Autodesk Inventor part; units mm, degrees
(part 2 of 2)
  spline S259 degree 2 poles (-78.2039, 3.4527) (-78.362, 3.5738) (-78.5473, 3.9615) (-78.5473, 4.2678) knots 0 0 0 1 2 2 2
  spline S260 degree 2 poles (-78.5473, 4.2678) (-78.5473, 4.5074) (-78.3842, 4.91) (-78.236, 5.0582) knots 0 0 0 1 2 2 2
  spline S261 degree 2 poles (-78.236, 5.0582) (-78.0878, 5.2064) (-77.6581, 5.3744) (-77.3938, 5.3744) knots 0 0 0 1 2 2 2
  spline S262 degree 2 poles (-77.3938, 5.3744) (-77.127, 5.3744) (-76.7145, 5.2262) (-76.5663, 5.0706) knots 0 0 0 1 2 2 2
  spline S263 degree 2 poles (-76.5663, 5.0706) (-76.3934, 4.8977) (-76.2156, 4.3493) (-76.2156, 3.9591) knots 0 0 0 1 2 2 2
  spline S264 degree 2 poles (-76.9739, 4.0727) (-76.9739, 4.3222) (-77.0579, 4.6433) (-77.1344, 4.7322) knots 0 0 0 1 2 2 2
  spline S265 degree 2 poles (-77.1344, 4.7322) (-77.1863, 4.7989) (-77.3197, 4.8557) (-77.3962, 4.8557) knots 0 0 0 1 2 2 2
  spline S266 degree 2 poles (-77.3962, 4.8557) (-77.4654, 4.8557) (-77.5938, 4.8014) (-77.6531, 4.7322) knots 0 0 0 1 2 2 2
  spline S267 degree 2 poles (-77.6531, 4.7322) (-77.705, 4.6729) (-77.7791, 4.4432) (-77.7791, 4.3074) knots 0 0 0 1 2 2 2
  spline S268 degree 2 poles (-77.7791, 4.3074) (-77.7791, 4.1592) (-77.7025, 3.969) (-77.6383, 3.9121) knots 0 0 0 1 2 2 2
  spline S269 degree 2 poles (-77.6383, 3.9121) (-77.5716, 3.8553) (-77.4061, 3.8109) (-77.3024, 3.8109) knots 0 0 0 1 2 2 2
  spline S270 degree 2 poles (-77.3024, 3.8109) (-77.2159, 3.8109) (-77.0356, 3.8578) (-76.9788, 3.8825) knots 0 0 0 1 2 2 2
  spline S271 degree 2 poles (-76.9788, 3.8825) (-76.9788, 3.9047) (-76.9739, 3.9887) (-76.9739, 4.0727) knots 0 0 0 1 2 2 2
  line L269 (-71.9276, 5.3126) -> (-72.9749, 2.2646)
  line L270 (-72.9749, 2.2646) -> (-73.7727, 2.2646)
  line L271 (-73.7727, 2.2646) -> (-74.82, 5.3126)
  line L272 (-74.82, 5.3126) -> (-74.0271, 5.3126)
  line L273 (-74.0271, 5.3126) -> (-73.3627, 3.2452)
  line L274 (-73.3627, 3.2452) -> (-72.7007, 5.3126)
  line L275 (-72.7007, 5.3126) -> (-71.9276, 5.3126)
  spline S272 degree 2 poles (-69.4798, 3.4132) (-69.4798, 2.8451) (-70.0998, 2.193) (-70.6654, 2.193) knots 0 0 0 1 2 2 2
  spline S273 degree 2 poles (-70.6654, 2.193) (-71.2286, 2.193) (-71.8535, 2.8451) (-71.8535, 3.4132) knots 0 0 0 1 2 2 2
  spline S274 degree 2 poles (-71.8535, 3.4132) (-71.8535, 3.9862) (-71.2286, 4.6359) (-70.6654, 4.6359) knots 0 0 0 1 2 2 2
  spline S275 degree 2 poles (-70.6654, 4.6359) (-70.1023, 4.6359) (-69.4798, 3.9838) (-69.4798, 3.4132) knots 0 0 0 1 2 2 2
  spline S276 degree 2 poles (-70.2134, 3.4083) (-70.2134, 3.6133) (-70.2801, 3.8874) (-70.3394, 3.969) knots 0 0 0 1 2 2 2
  spline S277 degree 2 poles (-70.3394, 3.969) (-70.4036, 4.0554) (-70.5642, 4.1221) (-70.6654, 4.1221) knots 0 0 0 1 2 2 2
  spline S278 degree 2 poles (-70.6654, 4.1221) (-70.7642, 4.1221) (-70.9199, 4.0628) (-70.9841, 3.9788) knots 0 0 0 1 2 2 2
  spline S279 degree 2 poles (-70.9841, 3.9788) (-71.0458, 3.8998) (-71.1199, 3.6207) (-71.1199, 3.4083) knots 0 0 0 1 2 2 2
  spline S280 degree 2 poles (-71.1199, 3.4083) (-71.1199, 3.1983) (-71.0508, 2.939) (-70.994, 2.8599) knots 0 0 0 1 2 2 2
  spline S281 degree 2 poles (-70.994, 2.8599) (-70.9372, 2.7809) (-70.7642, 2.7068) (-70.6605, 2.7068) knots 0 0 0 1 2 2 2
  spline S282 degree 2 poles (-70.6605, 2.7068) (-70.5741, 2.7068) (-70.3962, 2.7809) (-70.3419, 2.855) knots 0 0 0 1 2 2 2
  spline S283 degree 2 poles (-70.3419, 2.855) (-70.2801, 2.9414) (-70.2134, 3.1909) (-70.2134, 3.4083) knots 0 0 0 1 2 2 2
  line L276 (-68.3832, 2.2646) -> (-69.0995, 2.2646)
  line L277 (-69.0995, 2.2646) -> (-69.0995, 5.4485)
  line L278 (-69.0995, 5.4485) -> (-68.3832, 5.4485)
  line L279 (-68.3832, 5.4485) -> (-68.3832, 2.2646)
  spline S284 degree 2 poles (-66.9555, 2.2202) (-67.3927, 2.2202) (-67.7928, 2.5808) (-67.7928, 2.9908) knots 0 0 0 1 2 2 2
  line L280 (-67.7928, 2.9908) -> (-67.7928, 4.0653)
  line L281 (-67.7928, 4.0653) -> (-68.067, 4.0653)
  line L282 (-68.067, 4.0653) -> (-68.067, 4.5642)
  line L283 (-68.067, 4.5642) -> (-67.7928, 4.5642)
  line L284 (-67.7928, 4.5642) -> (-67.7928, 5.2213)
  line L285 (-67.7928, 5.2213) -> (-67.0765, 5.2213)
  line L286 (-67.0765, 5.2213) -> (-67.0765, 4.5642)
  line L287 (-67.0765, 4.5642) -> (-66.3849, 4.5642)
  line L288 (-66.3849, 4.5642) -> (-66.3849, 4.0653)
  line L289 (-66.3849, 4.0653) -> (-67.0765, 4.0653)
  line L290 (-67.0765, 4.0653) -> (-67.0765, 3.2477)
  spline S285 degree 2 poles (-67.0765, 3.2477) (-67.0765, 3.1267) (-67.0716, 2.9464) (-67.0419, 2.8747) knots 0 0 0 1 2 2 2
  spline S286 degree 2 poles (-67.0419, 2.8747) (-67.0123, 2.8031) (-66.8666, 2.7191) (-66.7282, 2.7191) knots 0 0 0 1 2 2 2
  spline S287 degree 2 poles (-66.7282, 2.7191) (-66.669, 2.7191) (-66.4837, 2.7685) (-66.4467, 2.7883) knots 0 0 0 1 2 2 2
  line L291 (-66.4467, 2.7883) -> (-66.3849, 2.7883)
  line L292 (-66.3849, 2.7883) -> (-66.3849, 2.2844)
  spline S288 degree 2 poles (-66.3849, 2.2844) (-66.501, 2.2548) (-66.7628, 2.2202) (-66.9555, 2.2202) knots 0 0 0 1 2 2 2
  spline S289 degree 2 poles (-77.5741, -1.8201) (-77.5741, -2.0474) (-77.747, -2.3907) (-77.8902, -2.5043) knots 0 0 0 1 2 2 2
  spline S290 degree 2 poles (-77.8902, -2.5043) (-78.0631, -2.6402) (-78.4732, -2.7538) (-78.7918, -2.7538) knots 0 0 0 1 2 2 2
  line L293 (-78.7918, -2.7538) -> (-80.0095, -2.7538)
  line L294 (-80.0095, -2.7538) -> (-80.0095, 0.2942)
  line L295 (-80.0095, 0.2942) -> (-78.9351, 0.2942)
  spline S291 degree 2 poles (-78.9351, 0.2942) (-78.5991, 0.2942) (-78.2533, 0.2423) (-78.1027, 0.1608) knots 0 0 0 1 2 2 2
  spline S292 degree 2 poles (-78.1027, 0.1608) (-77.9372, 0.0744) (-77.7766, -0.222) (-77.7766, -0.4147) knots 0 0 0 1 2 2 2
  spline S293 degree 2 poles (-77.7766, -0.4147) (-77.7766, -0.637) (-77.9989, -0.9853) (-78.1965, -1.0668) knots 0 0 0 1 2 2 2
  line L296 (-78.1965, -1.0668) -> (-78.1965, -1.0816)
  spline S294 degree 2 poles (-78.1965, -1.0816) (-77.9125, -1.1409) (-77.5741, -1.5089) (-77.5741, -1.8201) knots 0 0 0 1 2 2 2
  spline S295 degree 2 poles (-78.3645, -1.8078) (-78.3645, -1.6645) (-78.4781, -1.504) (-78.5917, -1.462) knots 0 0 0 1 2 2 2
  spline S296 degree 2 poles (-78.5917, -1.462) (-78.6609, -1.4348) (-78.9054, -1.4299) (-79.108, -1.4299) knots 0 0 0 1 2 2 2
  line L297 (-79.108, -1.4299) -> (-79.2488, -1.4299)
  line L298 (-79.2488, -1.4299) -> (-79.2488, -2.1981)
  line L299 (-79.2488, -2.1981) -> (-79.2068, -2.1981)
  spline S297 degree 2 poles (-79.2068, -2.1981) (-78.9104, -2.1981) (-78.6831, -2.1906) (-78.5646, -2.1388) knots 0 0 0 1 2 2 2
  spline S298 degree 2 poles (-78.5646, -2.1388) (-78.4608, -2.0918) (-78.3645, -1.9189) (-78.3645, -1.8078) knots 0 0 0 1 2 2 2
  spline S299 degree 2 poles (-78.5547, -0.5654) (-78.5547, -0.4913) (-78.6313, -0.3357) (-78.7103, -0.3011) knots 0 0 0 1 2 2 2
  spline S300 degree 2 poles (-78.7103, -0.3011) (-78.7844, -0.2665) (-78.9919, -0.2616) (-79.1969, -0.2616) knots 0 0 0 1 2 2 2
  line L300 (-79.1969, -0.2616) -> (-79.2488, -0.2616)
  line L301 (-79.2488, -0.2616) -> (-79.2488, -0.9087)
  line L302 (-79.2488, -0.9087) -> (-79.1524, -0.9087)
  spline S301 degree 2 poles (-79.1524, -0.9087) (-78.9573, -0.9087) (-78.7992, -0.9013) (-78.7152, -0.8618) knots 0 0 0 1 2 2 2
  spline S302 degree 2 poles (-78.7152, -0.8618) (-78.6238, -0.8173) (-78.5547, -0.6666) (-78.5547, -0.5654) knots 0 0 0 1 2 2 2
  spline S303 degree 2 poles (-75.9093, -2.5093) (-75.9834, -2.571) (-76.0995, -2.6698) (-76.1983, -2.7192) knots 0 0 0 1 2 2 2
  spline S304 degree 2 poles (-76.1983, -2.7192) (-76.2946, -2.7662) (-76.4774, -2.8156) (-76.6404, -2.8156) knots 0 0 0 1 2 2 2
  spline S305 degree 2 poles (-76.6404, -2.8156) (-76.9467, -2.8156) (-77.3493, -2.4055) (-77.3493, -2.0943) knots 0 0 0 1 2 2 2
  spline S306 degree 2 poles (-77.3493, -2.0943) (-77.3493, -1.8399) (-77.1443, -1.5237) (-76.9516, -1.4323) knots 0 0 0 1 2 2 2
  spline S307 degree 2 poles (-76.9516, -1.4323) (-76.7565, -1.3385) (-76.2156, -1.2644) (-75.9044, -1.2446) knots 0 0 0 1 2 2 2
  line L303 (-75.9044, -1.2446) -> (-75.9044, -1.2323)
  spline S308 degree 2 poles (-75.9044, -1.2323) (-75.9044, -1.0421) (-76.1859, -0.8964) (-76.4675, -0.8964) knots 0 0 0 1 2 2 2
  spline S309 degree 2 poles (-76.4675, -0.8964) (-76.5935, -0.8964) (-76.9343, -0.9877) (-77.0949, -1.0594) knots 0 0 0 1 2 2 2
  line L304 (-77.0949, -1.0594) -> (-77.1567, -1.0594)
  line L305 (-77.1567, -1.0594) -> (-77.1567, -0.5036)
  spline S310 degree 2 poles (-77.1567, -0.5036) (-77.0504, -0.474) (-76.5762, -0.39) (-76.3341, -0.39) knots 0 0 0 1 2 2 2
  spline S311 degree 2 poles (-76.3341, -0.39) (-75.7413, -0.39) (-75.1979, -0.7852) (-75.1979, -1.1903) knots 0 0 0 1 2 2 2
  line L306 (-75.1979, -1.1903) -> (-75.1979, -2.7538)
  line L307 (-75.1979, -2.7538) -> (-75.9093, -2.7538)
  line L308 (-75.9093, -2.7538) -> (-75.9093, -2.5093)
  line L309 (-75.9093, -2.1536) -> (-75.9093, -1.6769)
  spline S312 degree 2 poles (-75.9093, -1.6769) (-76.0921, -1.6942) (-76.3168, -1.7213) (-76.4255, -1.7609) knots 0 0 0 1 2 2 2
  spline S313 degree 2 poles (-76.4255, -1.7609) (-76.5219, -1.793) (-76.6256, -1.9263) (-76.6256, -2.035) knots 0 0 0 1 2 2 2
  spline S314 degree 2 poles (-76.6256, -2.035) (-76.6256, -2.1956) (-76.4502, -2.3166) (-76.2798, -2.3166) knots 0 0 0 1 2 2 2
  spline S315 degree 2 poles (-76.2798, -2.3166) (-76.1859, -2.3166) (-75.9883, -2.2302) (-75.9093, -2.1536) knots 0 0 0 1 2 2 2
  spline S316 degree 2 poles (-73.7875, -2.7983) (-74.2247, -2.7983) (-74.6249, -2.4376) (-74.6249, -2.0276) knots 0 0 0 1 2 2 2
  line L310 (-74.6249, -2.0276) -> (-74.6249, -0.9532)
  line L311 (-74.6249, -0.9532) -> (-74.8991, -0.9532)
  line L312 (-74.8991, -0.9532) -> (-74.8991, -0.4542)
  line L313 (-74.8991, -0.4542) -> (-74.6249, -0.4542)
  line L314 (-74.6249, -0.4542) -> (-74.6249, 0.2028)
  line L315 (-74.6249, 0.2028) -> (-73.9086, 0.2028)
  line L316 (-73.9086, 0.2028) -> (-73.9086, -0.4542)
  line L317 (-73.9086, -0.4542) -> (-73.217, -0.4542)
  line L318 (-73.217, -0.4542) -> (-73.217, -0.9532)
  line L319 (-73.217, -0.9532) -> (-73.9086, -0.9532)
  line L320 (-73.9086, -0.9532) -> (-73.9086, -1.7707)
  spline S317 degree 2 poles (-73.9086, -1.7707) (-73.9086, -1.8918) (-73.9036, -2.0721) (-73.874, -2.1437) knots 0 0 0 1 2 2 2
  spline S318 degree 2 poles (-73.874, -2.1437) (-73.8444, -2.2153) (-73.6986, -2.2993) (-73.5603, -2.2993) knots 0 0 0 1 2 2 2
  spline S319 degree 2 poles (-73.5603, -2.2993) (-73.501, -2.2993) (-73.3158, -2.2499) (-73.2787, -2.2302) knots 0 0 0 1 2 2 2
  line L321 (-73.2787, -2.2302) -> (-73.217, -2.2302)
  line L322 (-73.217, -2.2302) -> (-73.217, -2.734)
  spline S320 degree 2 poles (-73.217, -2.734) (-73.3331, -2.7637) (-73.5949, -2.7983) (-73.7875, -2.7983) knots 0 0 0 1 2 2 2
  spline S321 degree 2 poles (-72.0462, -2.7983) (-72.4834, -2.7983) (-72.8835, -2.4376) (-72.8835, -2.0276) knots 0 0 0 1 2 2 2
  line L323 (-72.8835, -2.0276) -> (-72.8835, -0.9532)
  line L324 (-72.8835, -0.9532) -> (-73.1577, -0.9532)
  line L325 (-73.1577, -0.9532) -> (-73.1577, -0.4542)
  line L326 (-73.1577, -0.4542) -> (-72.8835, -0.4542)
  line L327 (-72.8835, -0.4542) -> (-72.8835, 0.2028)
  line L328 (-72.8835, 0.2028) -> (-72.1672, 0.2028)
  line L329 (-72.1672, 0.2028) -> (-72.1672, -0.4542)
  line L330 (-72.1672, -0.4542) -> (-71.4756, -0.4542)
  line L331 (-71.4756, -0.4542) -> (-71.4756, -0.9532)
  line L332 (-71.4756, -0.9532) -> (-72.1672, -0.9532)
  line L333 (-72.1672, -0.9532) -> (-72.1672, -1.7707)
  spline S322 degree 2 poles (-72.1672, -1.7707) (-72.1672, -1.8918) (-72.1623, -2.0721) (-72.1326, -2.1437) knots 0 0 0 1 2 2 2
  spline S323 degree 2 poles (-72.1326, -2.1437) (-72.103, -2.2153) (-71.9573, -2.2993) (-71.8189, -2.2993) knots 0 0 0 1 2 2 2
  spline S324 degree 2 poles (-71.8189, -2.2993) (-71.7597, -2.2993) (-71.5744, -2.2499) (-71.5374, -2.2302) knots 0 0 0 1 2 2 2
  line L334 (-71.5374, -2.2302) -> (-71.4756, -2.2302)
  line L335 (-71.4756, -2.2302) -> (-71.4756, -2.734)
  spline S325 degree 2 poles (-71.4756, -2.734) (-71.5917, -2.7637) (-71.8535, -2.7983) (-72.0462, -2.7983) knots 0 0 0 1 2 2 2
  spline S326 degree 2 poles (-70.006, -2.8156) (-70.658, -2.8156) (-71.3521, -2.1931) (-71.3521, -1.6176) knots 0 0 0 1 2 2 2
  spline S327 degree 2 poles (-71.3521, -1.6176) (-71.3521, -1.0544) (-70.705, -0.3826) (-70.122, -0.3826) knots 0 0 0 1 2 2 2
  spline S328 degree 2 poles (-70.122, -0.3826) (-69.5959, -0.3826) (-69.0624, -0.9532) (-69.0624, -1.4817) knots 0 0 0 1 2 2 2
  line L336 (-69.0624, -1.4817) -> (-69.0624, -1.7411)
  line L337 (-69.0624, -1.7411) -> (-70.6358, -1.7411)
  spline S329 degree 2 poles (-70.6358, -1.7411) (-70.6259, -1.9016) (-70.5098, -2.1141) (-70.416, -2.1783) knots 0 0 0 1 2 2 2
  spline S330 degree 2 poles (-70.416, -2.1783) (-70.3246, -2.2425) (-70.0776, -2.2969) (-69.9319, -2.2969) knots 0 0 0 1 2 2 2
  spline S331 degree 2 poles (-69.9319, -2.2969) (-69.8084, -2.2969) (-69.5663, -2.2425) (-69.465, -2.1956) knots 0 0 0 1 2 2 2
  spline S332 degree 2 poles (-69.465, -2.1956) (-69.3761, -2.1585) (-69.2279, -2.0671) (-69.181, -2.0326) knots 0 0 0 1 2 2 2
  line L338 (-69.181, -2.0326) -> (-69.1044, -2.0326)
  line L339 (-69.1044, -2.0326) -> (-69.1044, -2.6254)
  spline S333 degree 2 poles (-69.1044, -2.6254) (-69.1933, -2.6599) (-69.3366, -2.7192) (-69.465, -2.7489) knots 0 0 0 1 2 2 2
  spline S334 degree 2 poles (-69.465, -2.7489) (-69.5811, -2.781) (-69.8281, -2.8156) (-70.006, -2.8156) knots 0 0 0 1 2 2 2
  spline S335 degree 2 poles (-69.7688, -1.3088) (-69.7738, -1.0816) (-69.9738, -0.842) (-70.1789, -0.842) knots 0 0 0 1 2 2 2
  spline S336 degree 2 poles (-70.1789, -0.842) (-70.3888, -0.842) (-70.6259, -1.094) (-70.6383, -1.3088) knots 0 0 0 1 2 2 2
  line L340 (-70.6383, -1.3088) -> (-69.7688, -1.3088)
  line L341 (-67.1506, -1.1335) -> (-67.2099, -1.1335)
  spline S337 degree 2 poles (-67.2099, -1.1335) (-67.2519, -1.1187) (-67.4075, -1.1038) (-67.5014, -1.1038) knots 0 0 0 1 2 2 2
  spline S338 degree 2 poles (-67.5014, -1.1038) (-67.6125, -1.1038) (-67.862, -1.1705) (-67.9781, -1.215) knots 0 0 0 1 2 2 2
  line L342 (-67.9781, -1.215) -> (-67.9781, -2.7538)
  line L343 (-67.9781, -2.7538) -> (-68.6944, -2.7538)
  line L344 (-68.6944, -2.7538) -> (-68.6944, -0.4542)
  line L345 (-68.6944, -0.4542) -> (-67.9781, -0.4542)
  line L346 (-67.9781, -0.4542) -> (-67.9781, -0.7852)
  spline S339 degree 2 poles (-67.9781, -0.7852) (-67.9287, -0.7407) (-67.7558, -0.6024) (-67.6841, -0.5604) knots 0 0 0 1 2 2 2
  spline S340 degree 2 poles (-67.6841, -0.5604) (-67.6051, -0.5135) (-67.3976, -0.4468) (-67.3062, -0.4468) knots 0 0 0 1 2 2 2
  spline S341 degree 2 poles (-67.3062, -0.4468) (-67.2716, -0.4468) (-67.1852, -0.4517) (-67.1506, -0.4542) knots 0 0 0 1 2 2 2
  line L347 (-67.1506, -0.4542) -> (-67.1506, -1.1335)
  line L348 (-64.7325, -0.4542) -> (-65.8909, -3.5961)
  line L349 (-65.8909, -3.5961) -> (-66.6616, -3.5961)
  line L350 (-66.6616, -3.5961) -> (-66.3133, -2.697)
  line L351 (-66.3133, -2.697) -> (-67.1556, -0.4542)
  line L352 (-67.1556, -0.4542) -> (-66.4047, -0.4542)
  line L353 (-66.4047, -0.4542) -> (-65.9205, -1.8967)
  line L354 (-65.9205, -1.8967) -> (-65.4685, -0.4542)
  line L355 (-65.4685, -0.4542) -> (-64.7325, -0.4542)
  dimension "d0" = 279.4
  dimension "d1" = 3.175
  dimension "d4" = 3.175
  dimension "d5" = 21.1667
  dimension "d29" = 6.35
  dimension "d30" = 6.35
  dimension "d31" = 11.1125
  dimension "d32" = 3.175
  dimension "d33" = 3.175
  dimension "d34" = 3.175
  dimension "d35" = 3.175
  dimension "d36" = 3.175
  dimension "d37" = 3.175
  dimension "d38" = 3.175
  dimension "d39" = 3.175
  dimension "d40" = 3.175
  dimension "d41" = 3.175
  dimension "d42" = 3.175
  dimension "d43" = 3.175
  dimension "d44" = 3.175
  dimension "d45" = 3.175
  dimension "d46" = 3.175
  dimension "d47" = 3.175
  dimension "d48" = 3.175
  dimension "d49" = 3.175
  dimension "d50" = 3.175
  dimension "d51" = 3.175
  dimension "d56" = 360
  dimension "d60" = 3.175
  dimension "d67" = 2.2606
  dimension "d70" = 360
  dimension "d74" = 139.7
  dimension "d75" = 50.8
  dimension "d76" = 107.95
  dimension "d77" = 63.5
  dimension "d84" = 8.4667
  dimension "d85" = 25.4
  dimension "d86" = 21.1667
  constraints: 51 centre point, 5 coincident, 70 other
  measures "d0" diameter of A0
  measures "d1" diameter of A1
  measures "d4" diameter of A2
  measures "d5" distance of A1.centre A2.centre
  measures "d29" diameter of A5
  measures "d30" diameter of A6
  measures "d31" vertical distance of A6.centre A5.centre
  measures "d32" diameter of A7
  measures "d33" diameter of A8
  measures "d34" diameter of A9
  measures "d35" diameter of A10
  measures "d36" diameter of A11
  measures "d37" diameter of A12
  measures "d38" diameter of A13
  measures "d39" diameter of A14
  measures "d40" diameter of A15
  measures "d41" diameter of A16
  measures "d42" diameter of A17
  measures "d43" diameter of A18
  measures "d44" diameter of A19
  measures "d45" diameter of A20
  measures "d46" diameter of A21
  measures "d47" diameter of A22
  measures "d48" diameter of A23
  measures "d49" diameter of A24
  measures "d50" diameter of A25
  measures "d51" diameter of A26
  measures "d60" diameter of A39
  measures "d67" diameter of A43
  measures "d74" distance of L8.start L8.end
  measures "d75" distance of L8.end L9.end
  measures "d76" distance of L12.start L12.end
  measures "d77" distance of L14.end L12.start
  measures "d84" vertical distance of A35.centre A43.centre
  measures "d85" horizontal distance of A35.centre point (0, 0)
  measures "d86" distance of A36.centre A35.centre
extrude "Extrusion4" add sketch "Sketch1" along normal blind 6.35 contours A0 | L16 L17 L18 L19 L20 L21 L22 L23 | L24 L25 L26 L27 | S0 S1 L28 L29 L30 S2 S3 S4 L31 S5 | S9 S8 L34 L33 L32 S7 S6 | S13 S12 L37 L36 L35 S11 S10 | L38 L39 L40 L41 | S14 S15 S16 S17 | S25 S24 S23 S22 S21 S20 S19 S18 | S26 S27 S28 S29 S30 L42 L43 S31 S32 S33 S34 S35 S36 L44 L45 S37 S38 | L46 L47 L48 L49 L50 L51 L52 L53 L54 L55 L56 L57 | L58 L59 L60 L61 L62 L63 L64 | L65 L66 L67 L68 | L69 L70 S39 S40 S41 S42 S43 L71 L72 S44 S45 S46 S47 L73 L74 | L75 L76 L77 L78 L79 L80 L81 | S48 S49 S50 S51 | S59 S58 S57 S56 S55 S54 S53 S52 | L82 L83 L84 L85 | S60 L86 L87 L88 L89 L90 L91 L92 L93 L94 L95 L96 S61 S62 S63 L97 L98 S64 | S65 S66 L99 L100 L101 S67 S68 S69 L102 S70 | S74 S73 L105 L104 L103 S72 S71 | S78 S77 L108 L107 L106 S76 S75 | S79 S80 S81 S82 S83 L109 S84 S85 L110 L111 S86 S87 L112 L113 L114 | S91 S90 S89 S88 L115 | S92 L116 L117 L118 L119 L120 L121 L122 L123 L124 L125 L126 S93 S94 S95 L127 L128 S96 | S97 L129 L130 L131 L132 L133 L134 L135 L136 L137 L138 L139 S98 S99 S100 L140 L141 S101 | S102 S103 S104 L142 L143 S105 S106 S107 S108 L144 L145 S109 S110 | L146 S112 S111 | L147 S113 S114 L148 L149 L150 L151 L152 S115 S116 S117 L157 L153 | L157 S117 L153 | L153 L158 L159 L160 L161 L154 L155 L156 L157 | L162 L163 L164 L165 L166 L167 L168 | S118 S119 S120 S121 | S129 S128 S127 S126 S125 S124 S123 S122 | L169 L170 L171 L172 | S130 L173 L174 L175 L176 L177 L178 L179 L180 L181 L182 L183 S131 S132 S133 L184 L185 S134 | S135 S136 S137 S138 S139 L186 S140 S141 L187 L188 S142 S143 L189 L190 L191 | S147 S146 S145 S144 L192 | S148 S149 S150 L193 L194 S151 S152 S153 S154 L195 S155 S156 S157 S158 S159 L196 L197 L198 | S164 S163 S162 S161 S160 L199 | S165 S166 S167 L200 L201 S168 S169 S170 S171 L202 L203 S172 S173 | L204 S175 S174 | L205 L206 L207 L208 L209 L210 L211 S176 S177 S178 L212 | S182 S181 L215 L214 L213 S180 S179 | S183 S184 S185 L216 L217 S186 S187 S188 S189 L218 L219 S190 S191 | L220 S193 S192 | S194 S195 S196 L221 L222 S197 S198 S199 S200 L223 S201 S202 S203 S204 S205 L224 L225 L226 | S210 S209 S208 S207 S206 L227 | L228 L229 S211 S212 L230 L231 L232 S213 S214 S215 L233 L234 L235 | L236 L237 L238 L239 | S216 S217 S218 S219 S220 L240 S221 S222 L241 L242 S223 S224 L243 L244 L245 | S228 S227 S226 S225 L246 | S229 L247 L248 L249 L250 L251 L252 L253 L254 L255 L256 L257 S230 S231 S232 L258 L259 S233 | S234 S235 S236 S237 | S245 S244 S243 S242 S241 S240 S239 S238 | L260 S246 S247 L261 L262 L263 L264 L265 S248 S249 S250 L266 | S251 S252 S253 L267 L268 S254 S255 S256 S257 S258 S259 S260 S261 S262 S263 | S271 S270 S269 S268 S267 S266 S265 S264 | L269 L270 L271 L272 L273 L274 L275 | S272 S273 S274 S275 | S283 S282 S281 S280 S279 S278 S277 S276 | L276 L277 L278 L279 | S284 L280 L281 L282 L283 L284 L285 L286 L287 L288 L289 L290 S285 S286 S287 L291 L292 S288 | S289 S290 L293 L294 L295 S291 S292 S293 L296 S294 | S298 S297 L299 L298 L297 S296 S295 | S302 S301 L302 L301 L300 S300 S299 | S303 S304 S305 S306 S307 L303 S308 S309 L304 L305 S310 S311 L306 L307 L308 | S315 S314 S313 S312 L309 | S316 L310 L311 L312 L313 L314 L315 L316 L317 L318 L319 L320 S317 S318 S319 L321 L322 S320 | S321 L323 L324 L325 L326 L327 L328 L329 L330 L331 L332 L333 S322 S323 S324 L334 L335 S325 | S326 S327 S328 L336 L337 S329 S330 S331 S332 L338 L339 S333 S334 | L340 S336 S335 | L341 S337 S338 L342 L343 L344 L345 L346 S339 S340 S341 L351 L347 | L351 S341 L347 | L347 L352 L353 L354 L355 L348 L349 L350 L351
extrude "Extrusion6" add sketch "Sketch1" along normal blind 6.604 contours L16 L17 L18 L19 L20 L21 L22 L23 | L24 L25 L26 L27 | S0 S1 L28 L29 L30 S2 S3 S4 L31 S5 | L38 L39 L40 L41 | S14 S15 S16 S17 | S26 S27 S28 S29 S30 L42 L43 S31 S32 S33 S34 S35 S36 L44 L45 S37 S38 | L46 L47 L48 L49 L50 L51 L52 L53 L54 L55 L56 L57 | L58 L59 L60 L61 L62 L63 L64 | L65 L66 L67 L68 | L69 L70 S39 S40 S41 S42 S43 L71 L72 S44 S45 S46 S47 L73 L74 | L75 L76 L77 L78 L79 L80 L81 | S48 S49 S50 S51 | L82 L83 L84 L85 | S60 L86 L87 L88 L89 L90 L91 L92 L93 L94 L95 L96 S61 S62 S63 L97 L98 S64 | S65 S66 L99 L100 L101 S67 S68 S69 L102 S70 | S79 S80 S81 S82 S83 L109 S84 S85 L110 L111 S86 S87 L112 L113 L114 | S92 L116 L117 L118 L119 L120 L121 L122 L123 L124 L125 L126 S93 S94 S95 L127 L128 S96 | S97 L129 L130 L131 L132 L133 L134 L135 L136 L137 L138 L139 S98 S99 S100 L140 L141 S101 | S102 S103 S104 L142 L143 S105 S106 S107 S108 L144 L145 S109 S110 | L147 S113 S114 L148 L149 L150 L151 L152 S115 S116 S117 L157 L153 | L157 S117 L153 | L153 L158 L159 L160 L161 L154 L155 L156 L157 | L162 L163 L164 L165 L166 L167 L168 | S118 S119 S120 S121 | L169 L170 L171 L172 | S130 L173 L174 L175 L176 L177 L178 L179 L180 L181 L182 L183 S131 S132 S133 L184 L185 S134 | S135 S136 S137 S138 S139 L186 S140 S141 L187 L188 S142 S143 L189 L190 L191 | S148 S149 S150 L193 L194 S151 S152 S153 S154 L195 S155 S156 S157 S158 S159 L196 L197 L198 | S165 S166 S167 L200 L201 S168 S169 S170 S171 L202 L203 S172 S173 | L205 L206 L207 L208 L209 L210 L211 S176 S177 S178 L212 | S183 S184 S185 L216 L217 S186 S187 S188 S189 L218 L219 S190 S191 | S194 S195 S196 L221 L222 S197 S198 S199 S200 L223 S201 S202 S203 S204 S205 L224 L225 L226 | L228 L229 S211 S212 L230 L231 L232 S213 S214 S215 L233 L234 L235 | L236 L237 L238 L239 | S216 S217 S218 S219 S220 L240 S221 S222 L241 L242 S223 S224 L243 L244 L245 | S229 L247 L248 L249 L250 L251 L252 L253 L254 L255 L256 L257 S230 S231 S232 L258 L259 S233 | S234 S235 S236 S237 | L260 S246 S247 L261 L262 L263 L264 L265 S248 S249 S250 L266 | S251 S252 S253 L267 L268 S254 S255 S256 S257 S258 S259 S260 S261 S262 S263 | L269 L270 L271 L272 L273 L274 L275 | S272 S273 S274 S275 | L276 L277 L278 L279 | S284 L280 L281 L282 L283 L284 L285 L286 L287 L288 L289 L290 S285 S286 S287 L291 L292 S288 | S289 S290 L293 L294 L295 S291 S292 S293 L296 S294 | S303 S304 S305 S306 S307 L303 S308 S309 L304 L305 S310 S311 L306 L307 L308 | S316 L310 L311 L312 L313 L314 L315 L316 L317 L318 L319 L320 S317 S318 S319 L321 L322 S320 | S321 L323 L324 L325 L326 L327 L328 L329 L330 L331 L332 L333 S322 S323 S324 L334 L335 S325 | S326 S327 S328 L336 L337 S329 S330 S331 S332 L338 L339 S333 S334 | L341 S337 S338 L342 L343 L344 L345 L346 S339 S340 S341 L351 L347 | L351 S341 L347 | L347 L352 L353 L354 L355 L348 L349 L350 L351
body "Solid4"
